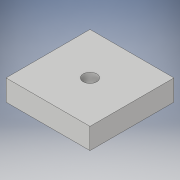
# Autodesk Inventor part: .25inAlluminumspacer-ver1-1111-2018
Saved by Autodesk Inventor 2017 (Build 210142000, 142)
## iProperties
Created: 2018-02-06
Part Number: .25inAlluminumspacer-ver1-1111-2018
Material: Generic
Document SubType Name: Modeling
Designer: Phyllis
Density: 1 g/cm^3
Appearance: Default
Author: Phyllis
Autodesk Inventor part; units mm, degrees
ref_plane "YZ Plane" through (0, 0, 0) normal (1, 0, 0) x (0, 1, 0)
ref_plane "XZ Plane" through (0, 0, 0) normal (0, 1, 0) x (-1, 0, 0)
ref_plane "XY Plane" through (0, 0, 0) normal (0, 0, 1) x (1, 0, 0)
sketch "Sketch1" plane through (0, 0, 0) normal (0, 1, 0) x (-1, 0, 0)
  line L0 (0, 0) -> (25.4, 0)
  line L1 (25.4, 0) -> (25.4, 25.4)
  line L2 (25.4, 25.4) -> (0, 25.4)
  line L3 (0, 25.4) -> (0, 0)
  dimension "d0" = 25.4
  dimension "d1" = 25.4
  constraints: 8 end point, 2 parallel, 1 horizontal, 1 perpendicular
  measures "d0" distance of L2.end L1.end
  measures "d1" distance of L1.end L0.end
extrude "Extrusion1" add sketch "Sketch1" along normal blind 6.35
sketch "Sketch2" plane through (0, 6.35, 0) normal (0, 1, 0) x (1, 0, 0)
  line L0 (-25.4, 0) -> (-25.4, -25.4) projected
  line L1 (0, 0) -> (-25.4, 0) projected
  point P0 (-12.7, -12.7)
  point P1 (-25.4, -12.7)
  point P2 (-12.7, 0)
  constraints: 2 midpoint, 1 horizontal alignment, 1 vertical alignment
hole "Hole1" at (-12.7, 6.35, 12.7) direction (0, -1, 0) diameter 4.1402 end through all
body "Solid1"
